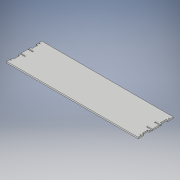
# Autodesk Inventor part: wall-front-scaled-model
Saved by Autodesk Inventor 2017 (Build 210142000, 142)
## iProperties
Created: 2017-02-28
Part Number: wall-front-scaled-model
Material: Generic
Document SubType Name: Modeling
Designer: John
Density: 1 g/cm^3
Appearance: Default
Author: John
Autodesk Inventor part; units mm, degrees
ref_plane "YZ Plane" through (0, 0, 0) normal (1, 0, 0) x (0, 1, 0)
ref_plane "XZ Plane" through (0, 0, 0) normal (0, 1, 0) x (-1, 0, 0)
ref_plane "XY Plane" through (0, 0, 0) normal (0, 0, 1) x (1, 0, 0)
sketch "Sketch1" plane through (0, 0, 0) normal (0, 1, 0) x (-1, 0, 0)
  line L0 (0, 0) -> (-280, 0)
  line L1 (-280, -75) -> (0, -75)
  line L2 (-280, -63) -> (-277, -63)
  line L3 (-277, -63) -> (-277, -51)
  line L4 (-277, -51) -> (-280, -51)
  line L5 (-280, -51) -> (-280, -63) construction
  line L6 (-280, -12) -> (-277, -12)
  line L7 (-277, -12) -> (-277, -24)
  line L8 (-277, -24) -> (-280, -24)
  line L9 (-280, -24) -> (-280, -12) construction
  line L10 (-140, 0) -> (-140, -75) construction
  line L11 (-280, -12) -> (-280, 0)
  line L12 (-280, -24) -> (-280, -28)
  line L13 (-280, -63) -> (-280, -75)
  circle A0 centre (-278, -7) radius 1
  line L14 (-278, -7) -> (-278, -12) construction
  line L15 (-278, -7) -> (-278, 0) construction
  circle A1 centre (-278, -68) radius 1
  line L16 (-280, -47) -> (-270, -47)
  line L17 (-270, -47) -> (-270, -45)
  line L18 (-270, -45) -> (-280, -45)
  line L19 (-280, -28) -> (-270, -28)
  line L20 (-270, -28) -> (-270, -30)
  line L21 (-270, -30) -> (-280, -30)
  line L22 (-280, -47) -> (-280, -51)
  line L23 (-280, -45) -> (-280, -47) construction
  line L24 (-280, -30) -> (-280, -45)
  line L25 (-280, -28) -> (-280, -30) construction
  line L26 (0, -63) -> (-3, -63)
  line L27 (-3, -63) -> (-3, -51)
  line L28 (-3, -51) -> (0, -51)
  line L29 (0, -51) -> (0, -63) construction
  line L30 (0, -12) -> (-3, -12)
  line L31 (-3, -12) -> (-3, -24)
  line L32 (-3, -24) -> (0, -24)
  line L33 (0, -24) -> (0, -12) construction
  line L34 (0, -12) -> (0, 0)
  line L35 (0, -24) -> (0, -28)
  line L36 (0, -63) -> (0, -75)
  circle A2 centre (-2, -7) radius 1
  line L37 (-2, -7) -> (-2, -12) construction
  line L38 (-2, -7) -> (-2, 0) construction
  circle A3 centre (-2, -68) radius 1
  line L39 (0, -47) -> (-10, -47)
  line L40 (-10, -47) -> (-10, -45)
  line L41 (-10, -45) -> (0, -45)
  line L42 (0, -28) -> (-10, -28)
  line L43 (-10, -28) -> (-10, -30)
  line L44 (-10, -30) -> (0, -30)
  line L45 (0, -47) -> (0, -51)
  line L46 (0, -45) -> (0, -47) construction
  line L47 (0, -30) -> (0, -45)
  line L48 (0, -28) -> (0, -30) construction
  dimension "d0" = 280
  dimension "d1" = 75
  dimension "d20" = 3
  dimension "d21" = 12
  dimension "d22" = 12
  dimension "d26" = 27
  dimension "d27" = 2
  dimension "d28" = 2
  dimension "d29" = 5
  dimension "d30" = 2
  dimension "d31" = 2
  dimension "d32" = 5
  dimension "d33" = 10
  dimension "d34" = 2
  dimension "d35" = 10
  dimension "d36" = 2
  dimension "d37" = 4
  constraints: 98 end point, 20 symmetric about line, 12 collinear, 8 parallel, 7 point on line, 5 horizontal, 5 perpendicular, 4 centre point, 2 midpoint, 1 vertical, 2 other
  measures "d0" distance of L1.end L1.start
  measures "d1" distance of L0.end L1.start
  measures "d20" distance of L4.end L3.end
  measures "d21" distance of L3.end L2.end
  measures "d22" distance of L6.end L7.end
  measures "d26" distance of L8.end L4.end
  measures "d27" diameter of A0
  measures "d28" distance from line of L11 L14.start
  measures "d29" distance of L14.start L14.end
  measures "d30" diameter of A1
  measures "d31" distance from line of L13 A1.centre
  measures "d32" distance from line of L2 A1.centre
  measures "d33" distance of L18.end L17.end
  measures "d34" distance of L17.end L16.end
  measures "d35" distance of L20.end L21.end
  measures "d36" distance of L19.end L20.end
  measures "d37" distance of L16.start L4.end
extrude "Extrusion2" add sketch "Sketch1" along normal blind 3
equation "\"d22\" = d21"
equation "\"d33\" = d35"
equation "\"d34\" = d36"
body "Solid2"
